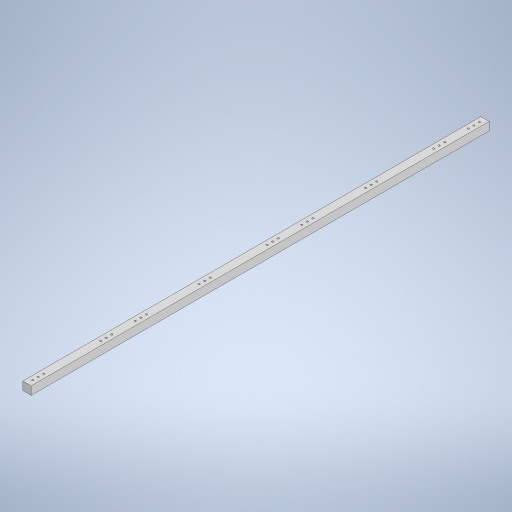
# Autodesk Inventor part: Part11
Saved by Autodesk Inventor 2023 (Build 270158000, 158)
## iProperties
Created: 2022-04-26
Part Number: Part11
Material: 一般
Document SubType Name: Modeling
Designer: yuta
Density: 1 g/cm^3
Appearance: 既定
Author: yuta
Autodesk Inventor part; units mm, degrees
ref_plane "YZ Plane" through (0, 0, 0) normal (1, 0, 0) x (0, 1, 0)
ref_plane "XZ Plane" through (0, 0, 0) normal (0, 1, 0) x (-1, 0, 0)
ref_plane "XY Plane" through (0, 0, 0) normal (0, 0, 1) x (1, 0, 0)
sketch "スケッチ1" plane through (0, 0, 0) normal (0, 0, 1) x (1, 0, 0)
  line L0 (0, 0) -> (15, 0)
  line L1 (15, 0) -> (15, 15)
  line L2 (15, 15) -> (0, 15)
  line L3 (0, 15) -> (0, 0)
  dimension "d0" = 15
  dimension "d1" = 15
  constraints: 8 end point, 2 parallel, 1 horizontal, 1 perpendicular
  measures "d0" distance of L2.end L1.end
  measures "d1" distance of L1.end L0.end
extrude "押し出し1" add sketch "スケッチ1" along normal blind 825
sketch "スケッチ2" plane through (0, 15, 825) normal (0, 1, 0) x (1, 0, 0)
  line L0 (15, 0) -> (0, 0) projected
  line L1 (15, 825) -> (15, 0) projected
  point P0 (0, 825)
  point P1 (7.5, 310)
  point P2 (7.5, 320)
  point P3 (7.5, 330)
  point P4 (7.5, 432.5)
  point P5 (7.5, 442.5)
  point P6 (7.5, 452.5)
  point P7 (7.5, 495)
  point P8 (7.5, 505)
  point P9 (7.5, 515)
  point P10 (7.5, 610)
  point P11 (7.5, 620)
  point P12 (7.5, 630)
  point P13 (7.5, 732.5)
  point P14 (7.5, 742.5)
  point P15 (7.5, 752.5)
  point P16 (7.5, 795)
  point P17 (7.5, 805)
  point P18 (7.5, 815)
  point P19 (7.5, 215)
  point P20 (7.5, 205)
  point P21 (7.5, 195)
  point P22 (7.5, 152.5)
  point P23 (7.5, 142.5)
  point P24 (7.5, 132.5)
  point P25 (7.5, 30)
  point P26 (7.5, 20)
  point P27 (7.5, 10)
  dimension "d4" = 310
  dimension "d5" = 7.5
  dimension "d6" = 10
  dimension "d7" = 10
  dimension "d8" = 102.5
  dimension "d9" = 10
  dimension "d10" = 10
  dimension "d11" = 42.5
  dimension "d12" = 10
  dimension "d13" = 10
  dimension "d14" = 95
  dimension "d15" = 10
  dimension "d16" = 10
  dimension "d17" = 102.5
  dimension "d18" = 10
  dimension "d19" = 10
  dimension "d20" = 42.5
  dimension "d21" = 10
  dimension "d22" = 10
  dimension "d23" = 95
  dimension "d24" = 10
  dimension "d25" = 10
  dimension "d26" = 42.5
  dimension "d27" = 10
  dimension "d28" = 10
  dimension "d29" = 102.5
  dimension "d30" = 10
  dimension "d31" = 10
  measures "d4" distance from line of L0 point (7.5, 310)
  measures "d5" distance from line of L1 point (7.5, 310)
  measures "d6" distance of point (7.5, 320) point (7.5, 310)
  measures "d7" distance of point (7.5, 330) point (7.5, 320)
  measures "d8" distance of point (7.5, 432.5) point (7.5, 330)
  measures "d9" distance of point (7.5, 442.5) point (7.5, 432.5)
  measures "d10" distance of point (7.5, 452.5) point (7.5, 442.5)
  measures "d11" distance of point (7.5, 452.5) point (7.5, 495)
  measures "d12" distance of point (7.5, 505) point (7.5, 495)
  measures "d13" distance of point (7.5, 515) point (7.5, 505)
  measures "d14" distance of point (7.5, 515) point (7.5, 610)
  measures "d15" distance of point (7.5, 610) point (7.5, 620)
  measures "d16" distance of point (7.5, 620) point (7.5, 630)
  measures "d17" distance of point (7.5, 630) point (7.5, 732.5)
  measures "d18" distance of point (7.5, 732.5) point (7.5, 742.5)
  measures "d19" distance of point (7.5, 742.5) point (7.5, 752.5)
  measures "d20" distance of point (7.5, 752.5) point (7.5, 795)
  measures "d21" distance of point (7.5, 795) point (7.5, 805)
  measures "d22" distance of point (7.5, 805) point (7.5, 815)
  measures "d23" distance of point (7.5, 310) point (7.5, 215)
  measures "d24" distance of point (7.5, 205) point (7.5, 215)
  measures "d25" distance of point (7.5, 195) point (7.5, 205)
  measures "d26" distance of point (7.5, 152.5) point (7.5, 195)
  measures "d27" distance of point (7.5, 142.5) point (7.5, 152.5)
  measures "d28" distance of point (7.5, 132.5) point (7.5, 142.5)
  measures "d29" distance of point (7.5, 30) point (7.5, 132.5)
  measures "d30" distance of point (7.5, 20) point (7.5, 30)
  measures "d31" distance of point (7.5, 10) point (7.5, 20)
hole "穴1" at (7.5, 15, 515) at (7.5, 15, 505) at (7.5, 15, 495) at (7.5, 15, 392.5) at (7.5, 15, 382.5) at (7.5, 15, 372.5) at (7.5, 15, 330) at (7.5, 15, 320) at (7.5, 15, 310) at (7.5, 15, 215) at (7.5, 15, 205) at (7.5, 15, 195) at (7.5, 15, 92.5) at (7.5, 15, 82.5) at (7.5, 15, 72.5) at (7.5, 15, 30) at (7.5, 15, 20) at (7.5, 15, 10) at (7.5, 15, 610) at (7.5, 15, 620) at (7.5, 15, 630) at (7.5, 15, 672.5) at (7.5, 15, 682.5) at (7.5, 15, 692.5) at (7.5, 15, 795) at (7.5, 15, 805) at (7.5, 15, 815) direction (0, -1, 0) diameter 3.2 end through all
